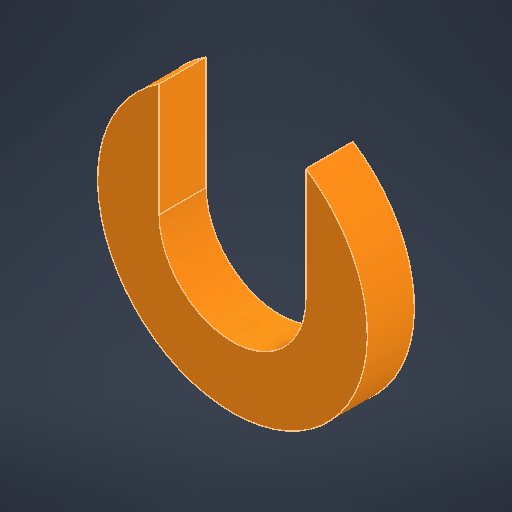
# Autodesk Inventor part: parça6
Saved by Autodesk Inventor 2025.4 (Build 294407000, 407)
## iProperties
Created: 2026-06-20
Part Number: parça6
Material: Generic
Document SubType Name: Modeling
Designer: yigithan
Density: 1 g/cm^3
Appearance: Orange
Author: yigithan
Autodesk Inventor part; units mm, degrees
ref_plane "YZ Plane" through (0, 0, 0) normal (1, 0, 0) x (0, 1, 0)
ref_plane "XZ Plane" through (0, 0, 0) normal (0, 1, 0) x (-1, 0, 0)
ref_plane "XY Plane" through (0, 0, 0) normal (0, 0, 1) x (1, 0, 0)
sketch "Sketch1" plane through (0, 0, 0) normal (0, 0, 1) x (1, 0, 0)
  circle A0 centre (0, 0) radius 4.96
  circle A1 centre (0, 0) radius 9.12
  line L0 (-4.96, 0) -> (-4.96, 7.6533)
  line L1 (4.96, 0) -> (4.96, 7.6533)
  dimension "d0" = 9.92
  dimension "d1" = 18.24
  constraints: 4 end point, 4 point on circle, 2 centre point, 2 coincident, 1 parallel, 1 tangent, 1 vertical
  measures "d0" diameter of A0
  measures "d1" diameter of A1
extrude "Extrusion1" add sketch "Sketch1" along normal blind 3.18 contours L1 A1 L0 A0 picked at (5.5376, 4.6162)
body "Solid1"
